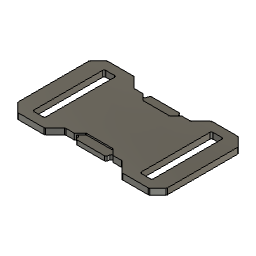
セス_バックル_mk1 v3 (Autodesk Fusion 360 design; units mm, degrees)
Autodesk Fusion 360 part; units mm, degrees
sketch "スケッチ1" plane through (0, 0, 0) normal (0, 0, 1) x (1, 0, 0)
  line L0 (50, 30) -> (-50, 30)
  line L1 (-50, 30) -> (-50, -30)
  line L2 (-50, -30) -> (50, -30)
  line L3 (50, -30) -> (50, 30)
  line L4 (50, 30) -> (-50, -30) construction
  line L5 (-50, 30) -> (50, -30) construction
  line L6 (-40, 24) -> (-32, 24)
  line L7 (-32, 24) -> (-32, -24)
  line L8 (-32, -24) -> (-40, -24)
  line L9 (-40, -24) -> (-40, 24)
  line L10 (-50, 0) -> (50, 0) construction
  line L11 (0, -30) -> (0, 30) construction
  line L12 (-50, 24) -> (-44, 30)
  line L13 (-26, 30) -> (-19, 23)
  line L14 (-19, 23) -> (-13, 23)
  line L15 (-13, 23) -> (-9, 19)
  line L16 (-50, -24) -> (-44, -30)
  line L17 (-26, -30) -> (-19, -23)
  line L18 (-19, -23) -> (-13, -23)
  line L19 (-13, -23) -> (-9, -19)
  line L20 (50, 24) -> (44, 30)
  line L21 (26, 30) -> (19, 23)
  line L22 (19, 23) -> (13, 23)
  line L23 (13, 23) -> (9, 19)
  line L24 (13, -23) -> (9, -19)
  line L25 (19, -23) -> (13, -23)
  line L26 (26, -30) -> (19, -23)
  line L27 (50, -24) -> (44, -30)
  line L28 (-9, 19) -> (9, 19)
  line L29 (-10, 25) -> (10, 25)
  line L30 (-10, 25) -> (-11, 21)
  line L31 (10, 25) -> (11, 21)
  line L32 (-10, -25) -> (-11, -21)
  line L33 (-10, -25) -> (10, -25)
  line L34 (10, -25) -> (11, -21)
  line L35 (-9, -19) -> (9, -19)
  line L36 (40, 24) -> (32, 24)
  line L37 (40, -24) -> (40, 24)
  line L38 (32, 24) -> (32, -24)
  line L39 (32, -24) -> (40, -24)
  dimension "d1" = 100
  dimension "d2" = 60
  dimension "d3" = 8
  dimension "d4" = 48
  dimension "d5" = 10
  dimension "d6" = 6
  dimension "d7" = 6
  dimension "d8" = 18
  dimension "d9" = 7
  dimension "d10" = 7
  dimension "d11" = 6
  dimension "d12" = 4
  dimension "d13" = 4
  dimension "d14" = 6
  dimension "d15" = 20
  constraint horizontal L0
  constraint perpendicular L0 L1
  constraint parallel L0 L2
  constraint parallel L1 L3
  constraint coincident L4 origin
  constraint coincident L5 origin
  constraint horizontal L6
  constraint vertical L7
  constraint horizontal L8
  constraint vertical L9
  constraint midpoint L1 L10.start
  constraint midpoint L3 L10.end
  constraint midpoint L2 L11.start
  constraint midpoint L0 L11.end
  constraint symmetric L6 L8 L10
  constraint coincident L1 L12.start
  constraint coincident L0 L12.end
  constraint coincident L0 L13.start
  constraint horizontal L14
  constraint symmetric L10 L12.start L16.start
  constraint symmetric L10 L12.end L16.end
  constraint symmetric L10 L13.start L17.start
  constraint symmetric L10 L13.end L17.end
  constraint symmetric L10 L14.end L18.end
  constraint symmetric L10 L15.end L19.end
  constraint symmetric L11 L12.start L20.start
  constraint symmetric L11 L12.end L20.end
  constraint symmetric L11 L13.start L21.start
  constraint symmetric L11 L13.end L21.end
  constraint symmetric L11 L14.end L22.end
  constraint symmetric L11 L15.end L23.end
  constraint symmetric L11 L16.start L27.start
  constraint symmetric L11 L16.end L27.end
  constraint symmetric L11 L17.start L26.start
  constraint symmetric L11 L17.end L25.start
  constraint symmetric L11 L18.end L24.start
  constraint symmetric L11 L19.end L24.end
  constraint perpendicular L11 L29
  constraint symmetric L11 L29.start L29.end
  constraint midpoint L15 L30.end
  constraint midpoint L23 L31.end
  constraint symmetric L10 L23.end L24.end
  constraint symmetric L10 L29.start L32.start
  constraint symmetric L10 L29.end L33.end
  constraint symmetric L10 L30.end L32.end
  constraint symmetric L10 L31.end L34.end
  constraint symmetric L6.start L11 L36.start
  constraint symmetric L6.end L11 L36.end
  constraint symmetric L7.end L11 L38.end
  constraint symmetric L8.end L11 L37.start
  measures "d1" distance of L1.end L2.end
  measures "d2" distance of L0.end L1.end
  measures "d3" distance of L6.start L6.end
  measures "d4" distance of L6.start L8.end
  measures "d5" distance of L1 L9
  measures "d6" distance of L0.end L12.start
  measures "d7" distance of L0.end L12.end
  measures "d8" distance of L12.end L13.start
  measures "d9" distance of L0 L13.end
  measures "d10" horizontal distance of L13.start L13.end
  measures "d11" distance of L13.end L14.end
  measures "d12" vertical distance of L14.end L15.end
  measures "d13" horizontal distance of L14.end L15.end
  measures "d14" distance of L28 L29
  measures "d15" distance of L29.start L29.end
extrude "押し出し1" add sketch "スケッチ1" along normal blind 4 contours L0 L1 L2 L3 L12 L13 L14 L15 L16 L17 L18 L19 L20 L21 L22 L23 L24 L25 L26 L27 L28 L35
extrude "押し出し2" add sketch "スケッチ1" along normal blind 3 contours L15 L23 L28 L29 L30 L31 | L19 L24 L32 L33 L34 L35
fillet "フィレット1" radius 1 16 edges at (-11, -21, 1.5) (-9, -19, 3.5) (11, -21, 1.5) (9, -19, 3.5) (11, 21, 1.5) (9, 19, 3.5) (-9, 19, 3.5) (-11, 21, 1.5) (32, -24, 2) (40, -24, 2) (-40, 24, 2) (-32, 24, 2) (40, 24, 2) (32, 24, 2) (-32, -24, 2) (-40, -24, 2)
fillet "フィレット2" radius 1 4 edges at (-19, -23, 2) (19, -23, 2) (19, 23, 2) (-19, 23, 2)
fillet "フィレット3" radius 1 12 edges at (-26, 30, 2) (-44, 30, 2) (-50, 24, 2) (-50, -24, 2) (-44, -30, 2) (-26, -30, 2) (26, -30, 2) (44, -30, 2) (50, -24, 2) (26, 30, 2) (44, 30, 2) (50, 24, 2)
fillet "フィレット4" radius 1 4 edges at (10, -25, 1.5) (-10, -25, 1.5) (-10, 25, 1.5) (10, 25, 1.5)
equation "d7 = d6"
